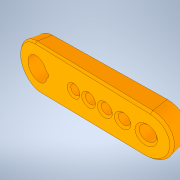
# Autodesk Inventor part: Рычаг натяжителя
Saved by Autodesk Inventor 2021.1 (Build 251245010, 245A)
## iProperties
Created: 2026-05-06
Part Number: Рычаг натяжителя
Material: Типовые
Document SubType Name: Modeling
Designer: Андрей Тарасов
Density: 1 g/cm^3
Appearance: По умолчанию
Author: Андрей Тарасов
Autodesk Inventor part; units mm, degrees
ref_plane "YZ Plane" through (0, 0, 0) normal (1, 0, 0) x (0, 1, 0)
ref_plane "XZ Plane" through (0, 0, 0) normal (0, 1, 0) x (-1, 0, 0)
ref_plane "XY Plane" through (0, 0, 0) normal (0, 0, 1) x (1, 0, 0)
sketch "Эскиз1" plane through (0, 0, 0) normal (0, 0, 1) x (1, 0, 0)
  arc A0 (3.8683, 1.1995) -> (3.8683, -1.1995) centre (0, 0) ccw
  circle A1 centre (14, 0) radius 1.6
  line L0 (-17.8, 0) -> (50.8, 0) construction
  circle A2 centre (0, 0) radius 8
  circle A3 centre (35, 0) radius 6
  circle A4 centre (35, 0) radius 2.1
  line L1 (0.4571, 7.9869) -> (35.3429, 5.9902)
  line L2 (0.4571, -7.9869) -> (35.3429, -5.9902)
  circle A5 centre (19, 0) radius 1.6
  circle A6 centre (24, 0) radius 1.6
  circle A7 centre (29, 0) radius 1.6
  arc A8 (4.3318, -0.695) -> (4.3318, 0.695) centre (4.05, 0) ccw
  arc A9 (4.05, 0) -> (3.8683, 1.1995) centre (0, 0) ccw construction
  arc A10 (3.8683, -1.1995) -> (4.05, 0) centre (0, 0) ccw construction
  arc A11 (3.8683, 1.1995) -> (4.3318, 0.695) centre (4.6324, 1.4364) ccw
  arc A12 (4.3318, -0.695) -> (3.8683, -1.1995) centre (4.6324, -1.4364) ccw
  dimension "d0" = 8.1
  dimension "d1" = 3.2
  dimension "d2" = 14
  dimension "d3" = 16
  dimension "d5" = 12
  dimension "d6" = 35
  dimension "d7" = 4.2
  dimension "d22" = 5
  dimension "d27" = 1.5
  dimension "d28" = 0.8
  constraints: 16 point on circle, 13 centre point, 8 tangent, 4 end point, 3 coincident, 3 point on line, 1 equal radius, 1 horizontal, 6 other
  measures "d0" diameter of A0
  measures "d1" diameter of A1
  measures "d2" distance of point (0, 0) A1.centre
  measures "d3" diameter of A2
  measures "d5" diameter of A3
  measures "d6" distance of A3.centre point (0, 0)
  measures "d7" diameter of A4
  measures "d22" distance of A1.centre A5.centre
  measures "d27" diameter of A8
  measures "d28" radius of A11
extrude "Выдавливание1" add sketch "Эскиз1" along normal blind 6 contours A2 | A2 L1 A3 A7 L2 | A3 A7 picked at (31.3752, 2.1355)
chamfer "Фаска1" distance 0.6 angle 45 22 edges at (17.9, -6.9886, 0) (41, 0, 0) (17.9, 6.9886, 0) (-8, 0, 0) (12.4, 0, 0) (32.9, 0, 0) (17.9, 6.9886, 6) (-8, 0, 6) (17.9, -6.9886, 6) (41, 0, 6) (12.4, 0, 6) (32.9, 0, 6) (17.4, 0, 6) (22.4, 0, 6) (27.4, 0, 6) (27.4, 0, 0) (22.4, 0, 0) (17.4, 0, 0) (-4.05, 0, 0) (4.0433, 0.8951, 0) (4.8, 0, 0) (4.0433, -0.8951, 0)
